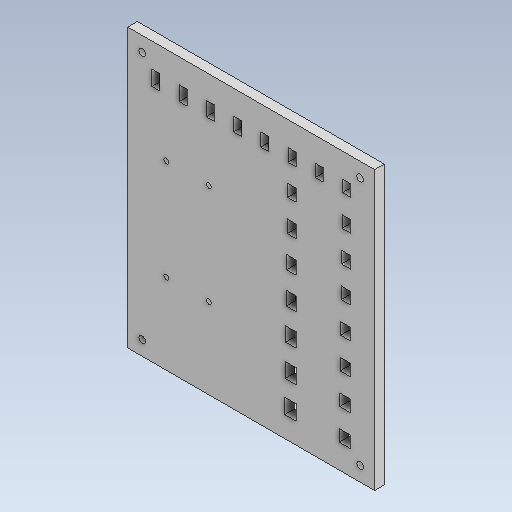
# Autodesk Inventor part: Board_Maria
Saved by Autodesk Inventor 2025.2 (Build 292293000, 293)
## iProperties
Created: 2025-02-22
Part Number: Board_Maria
Material: Generisch
Document SubType Name: Modeling
Designer: maria
Density: 1 g/cm^3
Appearance: Vorgabe
Author: maria
## iProperties of the stored document Board_Maria_3D-Druck.ipt
Created: 2025-04-29
Part Number: Board_Maria_3D-Druck
Material: Generisch
Document SubType Name: Modeling
Designer: maria
Density: 1 g/cm^3
Appearance: Vorgabe
Author: maria
Autodesk Inventor part; units mm, degrees
ref_plane "YZ Plane" through (0, 0, 0) normal (1, 0, 0) x (0, 1, 0)
ref_plane "XZ Plane" through (0, 0, 0) normal (0, 1, 0) x (-1, 0, 0)
ref_plane "XY Plane" through (0, 0, 0) normal (0, 0, 1) x (1, 0, 0)
sketch "Skizze1" plane through (0, 0, 0) normal (0, 1, 0) x (-1, 0, 0)
  line L0 (0, 0) -> (255.6, 0)
  line L1 (255.6, 0) -> (255.6, -287.6)
  line L2 (255.6, -287.6) -> (0, -287.6)
  line L3 (0, -287.6) -> (0, 0)
  dimension "d0" = 287.6
  dimension "d1" = 255.6
  constraints: 8 end point, 2 parallel, 1 horizontal, 1 perpendicular
  measures "d0" distance of L0.end L1.end
  measures "d1" distance of L1.end L2.end
extrude "Extrusion1" add sketch "Skizze1" along normal blind 10
sketch "Skizze4" plane through (0, 10, 0) normal (0, 1, 0) x (1, 0, 0)
  line L0 (-25, 25) -> (-33.2, 25)
  line L1 (-33.2, 25) -> (-33.2, 37.2)
  line L2 (-33.2, 37.2) -> (-25, 37.2)
  line L3 (-25, 37.2) -> (-25, 25)
  line L4 (-109.6, 25) -> (-117.8, 25)
  line L5 (-117.8, 25) -> (-117.8, 38.7)
  line L6 (-117.8, 38.7) -> (-109.6, 38.7)
  line L7 (-109.6, 38.7) -> (-109.6, 25)
  line L8 (-137.8, 25) -> (-146, 25)
  line L9 (-146, 25) -> (-146, 39.2)
  line L10 (-146, 39.2) -> (-137.8, 39.2)
  line L11 (-137.8, 39.2) -> (-137.8, 25)
  line L12 (-166, 39.7) -> (-166, 25)
  line L13 (-222.4, 25) -> (-230.6, 25)
  line L14 (-230.6, 25) -> (-230.6, 40.7)
  line L15 (-25, 57.2) -> (-33.7, 57.2)
  line L16 (-33.7, 57.2) -> (-33.7, 69.4)
  line L17 (-33.7, 69.4) -> (-25, 69.4)
  line L18 (-25, 69.4) -> (-25, 57.2)
  line L19 (-25, 89.4) -> (-34.2, 89.4)
  line L20 (-34.2, 89.4) -> (-34.2, 101.6)
  line L21 (-34.2, 101.6) -> (-25, 101.6)
  line L22 (-25, 101.6) -> (-25, 89.4)
  line L23 (-25, 121.6) -> (-34.7, 121.6)
  line L24 (-34.7, 121.6) -> (-34.7, 133.8)
  line L25 (-34.7, 133.8) -> (-25, 133.8)
  line L26 (-25, 133.8) -> (-25, 121.6)
  line L27 (-25, 153.8) -> (-35.2, 153.8)
  line L28 (-35.2, 153.8) -> (-35.2, 166)
  line L29 (-35.2, 166) -> (-25, 166)
  line L30 (-25, 166) -> (-25, 153.8)
  line L31 (-25, 186) -> (-35.7, 186)
  line L32 (-35.7, 186) -> (-35.7, 198.2)
  line L33 (-35.7, 198.2) -> (-25, 198.2)
  line L34 (-25, 198.2) -> (-25, 186)
  line L35 (-25, 230.4) -> (-25, 218.2)
  line L36 (-222.4, 25) -> (-222.4, 38.5)
  line L37 (-222.4, 38.5) -> (-222.4, 40.7)
  line L38 (-230.6, 40.7) -> (-222.4, 40.7)
  line L39 (-25, 218.2) -> (-36.2, 218.2)
  line L40 (-36.2, 218.2) -> (-36.2, 230.4)
  line L41 (-36.2, 230.4) -> (-25, 230.4)
  line L42 (-25, 250.4) -> (-25, 262.6)
  line L43 (-25, 262.6) -> (-36.7, 262.6)
  line L44 (-36.7, 262.6) -> (-36.7, 250.4)
  line L45 (-36.7, 250.4) -> (-25, 250.4)
  line L46 (-53.2, 25) -> (-61.4, 25)
  line L47 (-61.4, 25) -> (-61.4, 37.7)
  line L48 (-61.4, 37.7) -> (-53.2, 37.7)
  line L49 (-53.2, 37.7) -> (-53.2, 25)
  line L50 (-89.6, 25) -> (-89.6, 37.7)
  line L51 (-89.6, 37.7) -> (-89.6, 38.2)
  line L52 (0, 0) -> (0, 287.6) projected
  line L53 (-255.6, 0) -> (0, 0) projected
  line L54 (-81.4, 69.9) -> (-90.1, 69.9)
  line L55 (-90.1, 69.9) -> (-90.1, 57.2)
  line L56 (-90.1, 57.2) -> (-81.4, 57.2)
  line L57 (-81.4, 102.6) -> (-90.6, 102.6)
  line L58 (-90.6, 102.6) -> (-90.6, 89.4)
  line L59 (-90.6, 89.4) -> (-81.4, 89.4)
  line L60 (-81.4, 121.6) -> (-81.4, 135.3)
  line L61 (-81.4, 135.3) -> (-91.1, 135.3)
  line L62 (-91.1, 135.3) -> (-91.1, 121.6)
  line L63 (-91.1, 121.6) -> (-81.4, 121.6)
  line L64 (-81.4, 153.8) -> (-81.4, 168)
  line L65 (-81.4, 168) -> (-91.6, 168)
  line L66 (-91.6, 168) -> (-91.6, 153.8)
  line L67 (-91.6, 153.8) -> (-81.4, 153.8)
  line L68 (-81.4, 186) -> (-81.4, 200.7)
  line L69 (-81.4, 200.7) -> (-92.1, 200.7)
  line L70 (-92.1, 200.7) -> (-92.1, 186)
  line L71 (-92.1, 186) -> (-81.4, 186)
  line L72 (-81.4, 218.2) -> (-81.4, 233.4)
  line L73 (-81.4, 233.4) -> (-92.6, 233.4)
  line L74 (-92.6, 233.4) -> (-92.6, 218.2)
  line L75 (-92.6, 218.2) -> (-81.4, 218.2)
  line L76 (-81.4, 250.4) -> (-81.4, 266.1)
  line L77 (-81.4, 266.1) -> (-93.1, 266.1)
  line L78 (-93.1, 266.1) -> (-93.1, 250.4)
  line L79 (-93.1, 250.4) -> (-81.4, 250.4)
  line L80 (-194.2, 25) -> (-202.4, 25)
  line L81 (-202.4, 25) -> (-202.4, 40.2)
  line L82 (-202.4, 40.2) -> (-194.2, 40.2)
  line L83 (-194.2, 40.2) -> (-194.2, 25)
  line L84 (-166, 25) -> (-174.2, 25)
  line L85 (-166, 39.7) -> (-174.2, 39.7)
  line L86 (-174.2, 39.7) -> (-174.2, 25)
  line L87 (-166, 25) -> (-174.2, 25)
  line L88 (-81.4, 25) -> (-89.6, 25)
  line L89 (-81.4, 25) -> (-81.4, 38.2)
  line L90 (-81.4, 38.2) -> (-89.6, 38.2)
  line L91 (-202.4, 25) -> (-194.2, 25)
  line L92 (-174.2, 25) -> (-166, 25)
  line L93 (-146, 25) -> (-137.8, 25)
  line L94 (-137.8, 25) -> (-146, 25)
  line L95 (-109.6, 25) -> (-117.8, 25)
  line L96 (-81.4, 25) -> (-89.6, 25)
  line L97 (-25, 25) -> (-33.2, 25)
  line L98 (-53.2, 25) -> (-61.4, 25)
  line L99 (-166, 25) -> (-174.2, 25)
  line L100 (-194.2, 25) -> (-202.4, 25)
  line L101 (-222.4, 25) -> (-230.6, 25)
  line L102 (-25, 57.2) -> (-33.7, 57.2)
  line L103 (-81.4, 57.2) -> (-90.1, 57.2)
  line L104 (-25, 89.4) -> (-34.2, 89.4)
  line L105 (-81.4, 89.4) -> (-90.6, 89.4)
  line L106 (-25, 121.6) -> (-34.7, 121.6)
  line L107 (-81.4, 121.6) -> (-91.1, 121.6)
  line L108 (-25, 153.8) -> (-35.2, 153.8)
  line L109 (-81.4, 153.8) -> (-91.6, 153.8)
  line L110 (-25, 186) -> (-35.7, 186)
  line L111 (-81.4, 186) -> (-92.1, 186)
  line L112 (-25, 218.2) -> (-36.2, 218.2)
  line L113 (-81.4, 218.2) -> (-92.6, 218.2)
  line L114 (-25, 250.4) -> (-36.7, 250.4)
  line L115 (-81.4, 250.4) -> (-93.1, 250.4)
  line L116 (-81.4, 26.1) -> (-81.4, 294.0046)
  line L117 (-81.4, 69.9) -> (-81.4, 47.2)
  line L118 (-90.1, 57.2) -> (-90.1, 69.9)
  line L119 (-81.4, 89.4) -> (-81.4, 102.6)
  line L120 (-90.6, 102.6) -> (-90.6, 89.4)
  line L121 (-25, 25) -> (-25, 285.2671)
  line L122 (-25, 25) -> (-258.6914, 25)
  line L123 (0, 287.6) -> (-255.6, 287.6) projected
  line L124 (-255.6, 287.6) -> (-255.6, 0) projected
  point P0 (-29.6, 89.4)
  point P1 (-29.35, 69.4)
  point P2 (-29.85, 121.6)
  point P3 (-29.6, 101.6)
  point P4 (-30.1, 153.8)
  point P5 (-29.85, 133.8)
  point P6 (-30.35, 186)
  point P7 (-30.1, 166)
  point P8 (-30.6, 218.2)
  point P9 (-30.35, 198.2)
  point P10 (-30.85, 250.4)
  point P11 (-30.6, 230.4)
  point P12 (-81.4, 25)
  point P13 (-53.2, 31.35)
  point P14 (-61.4, 31.35)
  point P15 (-109.6, 31.85)
  point P16 (-137.8, 32.1)
  point P17 (-117.8, 31.85)
  point P18 (-166, 27.1)
  point P19 (-146, 32.1)
  point P20 (-169.2, 27.6)
  point P21 (-222.4, 31.75)
  point P22 (-25, 31.1)
  point P23 (-29.1, 25)
  point P24 (-29.35, 57.2)
  point P25 (-85.75, 57.2)
  point P26 (-86.25, 121.6)
  point P27 (-141.9, 25)
  point P28 (-86.5, 153.8)
  point P29 (-86.75, 186)
  point P30 (-87, 218.2)
  point P31 (-81.4, 225.8)
  point P32 (-81.4, 258.25)
  point P33 (-226.5, 40.7)
  point P34 (-86, 102.6)
  point P35 (-86.25, 135.3)
  point P36 (-86.75, 200.7)
  point P37 (-87.25, 250.4)
  point P38 (-87, 233.4)
  point P39 (-86, 89.4)
  point P40 (-85.75, 69.9)
  point P41 (-86.5, 168)
  point P42 (-33.7, 63.3)
  point P43 (-80, 91)
  point P44 (-34.2, 95.5)
  point P45 (-81.4, 128.45)
  point P46 (-34.7, 127.7)
  point P47 (-81.4, 160.9)
  point P48 (-35.2, 159.9)
  point P49 (-81.4, 193.35)
  point P50 (-35.7, 192.1)
  point P51 (-36.2, 224.3)
  point P52 (-36.7, 256.5)
  point P53 (-81.4, 58.55)
  point P54 (-76, 52.7)
  point P55 (-76, 65.4)
  point P56 (-25, 256.5)
  point P57 (-57.3, 25)
  point P58 (-29.6, 89.4)
  point P59 (-86, 89.4)
  point P60 (-87, 218.2)
  point P61 (-30.6, 218.2)
  point P62 (-87.25, 250.4)
  point P63 (-30.85, 250.4)
  point P64 (-85.75, 57.2)
  point P65 (-85.5, 38.2)
  point P66 (-29.35, 57.2)
  point P67 (-30.35, 186)
  point P68 (-87.25, 266.1)
  point P69 (-30.85, 262.6)
  point P70 (-230.6, 32.85)
  point P71 (-81.4, 31.6)
  point P72 (-226.5, 25)
  dimension "d10" = 8.2
  dimension "d11" = 12.2
  dimension "d17" = 12.2
  dimension "d18" = 9.2
  dimension "d19" = 12.2
  dimension "d20" = 9.7
  dimension "d21" = 12.2
  dimension "d22" = 10.2
  dimension "d23" = 12.2
  dimension "d24" = 10.7
  dimension "d25" = 12.2
  dimension "d27" = 12.2
  dimension "d29" = 13.7
  dimension "d30" = 14.2
  dimension "d32" = 14.7
  dimension "d53" = 11.2
  dimension "d60" = 12.2
  dimension "d61" = 11.7
  dimension "d64" = 12.7
  dimension "d65" = 8.2
  dimension "d79" = 12.7
  dimension "d80" = 13.2
  dimension "d81" = 9.2
  dimension "d82" = 13.7
  dimension "d83" = 9.7
  dimension "d84" = 14.2
  dimension "d85" = 10.2
  dimension "d86" = 14.7
  dimension "d87" = 10.7
  dimension "d88" = 15.2
  dimension "d89" = 11.2
  dimension "d90" = 15.7
  dimension "d91" = 11.7
  dimension "d149" = 15.7
  dimension "d152" = 8.2
  dimension "d153" = 8.2
  dimension "d155" = 20
  dimension "d156" = 8.2
  dimension "d159" = 20
  dimension "d160" = 20
  dimension "d162" = 20
  dimension "d163" = 20
  dimension "d164" = 20
  dimension "d165" = 20
  dimension "d166" = 20
  dimension "d167" = 20
  dimension "d168" = 20
  dimension "d169" = 20
  dimension "d187" = 19
  dimension "d188" = 18.5
  dimension "d189" = 18
  dimension "d191" = 17.5
  dimension "d197" = 8.2
  dimension "d198" = 15.2
  dimension "d199" = 20
  dimension "d200" = 8.2
  dimension "d201" = 20
  dimension "d203" = 8.2
  dimension "d205" = 13.2
  dimension "d207" = 8.7
  dimension "d209" = 45.8
  dimension "d219" = 8.7
  dimension "d239" = 0
  dimension "d240" = 0
  constraints: 240 end point, 67 midpoint, 43 perpendicular, 39 horizontal, 26 collinear, 21 parallel, 19 point on line, 10 vertical, 13 other
  measures "d10" distance of L0.start L0.end
  measures "d11" distance of L2.end L0.start
  measures "d17" distance of L17.end L15.start
  measures "d18" distance of L19.start L19.end
  measures "d19" distance of L21.end L19.start
  measures "d20" distance of L23.start L23.end
  measures "d21" distance of L25.end L23.start
  measures "d22" distance of L27.start L27.end
  measures "d23" distance of L29.end L27.start
  measures "d24" distance of L31.start L31.end
  measures "d25" distance of L33.end L31.start
  measures "d27" distance of L35.start L35.end
  measures "d29" distance of L6.end L4.start
  measures "d30" distance of L10.end L8.start
  measures "d32" distance of L12.start L12.end
  measures "d53" distance of L35.end L39.end
  measures "d60" distance of L42.start L42.end
  measures "d61" distance of L44.end L42.start
  measures "d64" distance of L48.end L46.start
  measures "d65" distance of L46.start L46.end
  measures "d79" distance of L54.start L56.end
  measures "d80" distance of L59.end L57.start
  measures "d81" distance of L59.end L58.end
  measures "d82" distance of L60.start L60.end
  measures "d83" distance of L62.end L60.start
  measures "d84" distance of L64.start L64.end
  measures "d85" distance of L66.end L64.start
  measures "d86" distance of L68.start L68.end
  measures "d87" distance of L70.end L68.start
  measures "d88" distance of L72.start L72.end
  measures "d89" distance of L74.end L72.start
  measures "d90" distance of L76.start L76.end
  measures "d91" distance of L78.end L76.start
  measures "d149" distance from line of point (-226.5, 40.7) L13
  measures "d152" distance of L4.start L4.end
  measures "d153" distance of L8.start L8.end
  measures "d155" distance between parallel lines of L7 L50
  measures "d156" distance of L13.end L13.start
  measures "d159" distance between parallel lines of L12 L9
  measures "d160" distance between parallel lines of L11 L5
  measures "d162" distance between parallel lines of L49 L1
  measures "d163" distance from line of L35.start L45
  measures "d164" distance of L33.end L35.end
  measures "d165" distance from line of point (-30.1, 166) L31
  measures "d166" distance of L25.end L27.start
  measures "d167" distance of L21.end L23.start
  measures "d168" distance of L17.end L19.start
  measures "d169" distance of L2.end L15.start
  measures "d187" vertical distance of point (-86.25, 121.6) point (-86, 102.6)
  measures "d188" vertical distance of point (-86.5, 153.8) point (-86.25, 135.3)
  measures "d189" vertical distance of point (-86.75, 186) point (-86.5, 168)
  measures "d191" vertical distance of point (-87, 218.2) point (-86.75, 200.7)
  measures "d197" distance between parallel lines of L81 L83
  measures "d198" distance of L82.end L80.start
  measures "d199" distance between parallel lines of L36 L81
  measures "d200" distance between parallel lines of L86 L12
  measures "d201" distance between parallel lines of L83 L86
  measures "d203" distance of L88.start L50.start
  measures "d205" distance of L88.start L89.end
  measures "d207" distance of L15.start L15.end
  measures "d209" horizontal distance of point (-80, 91) point (-34.2, 95.5)
  measures "d239" vertical distance of point (-87, 218.2) point (-30.6, 218.2)
  measures "d240" vertical distance of point (-87.25, 250.4) point (-30.85, 250.4)
extrude "Extrusion4" cut sketch "Skizze4" against normal blind 30 contours L88 L50 L51 L90 L89 | L46 L47 L48 L49 | L45 L44 L43 L42 | L39 L40 L41 L35 | L31 L32 L33 L34 | L27 L28 L29 L30 | L23 L24 L25 L26 | L19 L20 L21 L22 | L15 L16 L17 L18 | L0 L1 L2 L3 | L4 L5 L6 L7 | L8 L9 L10 L11 | L56 L55 L54 L116 | L84 L86 L85 L12 | L59 L58 L57 L116 | L80 L81 L82 L83 | L63 L62 L61 L60 | L13 L14 L38 L37 L36 | L67 L66 L65 L64 | L71 L70 L69 L68 | L75 L74 L73 L72 | L76 L79 L78 L77
sketch "Skizze5" plane through (0, 10, 0) normal (0, 1, 0) x (1, 0, 0)
  circle A0 centre (-215.6, 100) radius 2.5
  circle A1 centre (-215.6, 204) radius 2.5
  line L0 (-255.6, 0) -> (0, 0) projected
  line L1 (-255.6, 287.6) -> (-255.6, 0) projected
  circle A2 centre (-171.6, 100) radius 2.5
  circle A3 centre (-171.6, 204) radius 2.5
  line L2 (-171.6, 100) -> (-215.6, 100)
  line L3 (-215.6, 100) -> (-215.6, 204)
  line L4 (-215.6, 204) -> (-171.6, 204)
  line L5 (-171.6, 204) -> (-171.6, 100)
  dimension "d110" = 5
  dimension "d116" = 5
  dimension "d119" = 100
  dimension "d224" = 5
  dimension "d225" = 5
  dimension "d230" = 104
  dimension "d231" = 44
  dimension "d233" = 40
  dimension "d234" = 0
  constraints: 8 end point, 4 centre point, 2 parallel, 1 horizontal, 1 perpendicular
  measures "d110" diameter of A0
  measures "d116" diameter of A1
  measures "d119" distance from line of A0.centre L0
  measures "d224" diameter of A2
  measures "d225" diameter of A3
  measures "d230" distance of A3.centre L2.start
  measures "d231" distance of L3.end A3.centre
  measures "d233" distance from line of L1 A0.centre
  measures "d234" distance of A0.centre L2.end
extrude "Extrusion5" cut sketch "Skizze5" against normal blind 30 contours L2 L3 A0 | A0 L3 L2 | L2 L5 A2 | A2 L5 L2 | L3 L4 A1 | A1 L4 L3 | L5 L4 A3 | A3 L4 L5
sketch "Skizze6" plane through (0, 0, 0) normal (0, -1, 0) x (1, 0, 0)
  line L0 (-255.6, -287.6) -> (-255.6, 0) projected
  line L1 (-255.6, 0) -> (0, 0) projected
  line L2 (0, 0) -> (0, -287.6) projected
  line L3 (0, -287.6) -> (-255.6, -287.6) projected
  point P0 (-240.6, -15)
  point P1 (-240.6, -272.6)
  point P2 (-15, -272.6)
  point P3 (-15, -15)
  dimension "d265" = 15
  dimension "d266" = 15
  dimension "d267" = 15
  dimension "d268" = 15
  dimension "d269" = 15
  dimension "d270" = 15
  dimension "d271" = 15
  dimension "d272" = 15
  measures "d265" distance from line of L0 point (-240.6, -15)
  measures "d266" distance from line of L1 point (-240.6, -15)
  measures "d267" distance from line of point (-15, -15) L1
  measures "d268" distance from line of L2 point (-15, -15)
  measures "d269" distance from line of L3 point (-15, -272.6)
  measures "d270" distance from line of point (-15, -272.6) L2
  measures "d271" distance from line of point (-240.6, -272.6) L3
  measures "d272" distance from line of L0 point (-240.6, -272.6)
hole "Bohrung1" at (-240.6, 0, -15) at (-240.6, 0, -272.6) at (-15, 0, -272.6) at (-15, 0, -15) direction (0, 1, 0) diameter 7 depth 10
